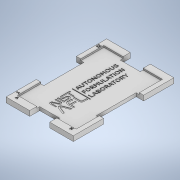
# Autodesk Inventor part: Thermal_underplate
Saved by Autodesk Inventor 2020 (Build 240168000, 168)
## iProperties
Created: 2021-08-09
Part Number: Thermal_underplate
Material: Generic
Document SubType Name: Modeling
Designer: pab2
Density: 1 g/cm^3
Appearance: Default
Author: pab2
Autodesk Inventor part; units mm, degrees
(part 1 of 3)
ref_plane "YZ Plane" through (0, 0, 0) normal (1, 0, 0) x (0, 1, 0)
ref_plane "XZ Plane" through (0, 0, 0) normal (0, 1, 0) x (-1, 0, 0)
ref_plane "XY Plane" through (0, 0, 0) normal (0, 0, 1) x (1, 0, 0)
sketch "Sketch1" plane through (0, 0, 0) normal (0, 1, 0) x (-1, 0, 0)
  line L0 (0, 0) -> (85.48, 0)
  line L1 (85.48, 0) -> (85.48, -127.76)
  line L2 (85.48, -127.76) -> (0, -127.76)
  line L3 (0, -127.76) -> (0, 0)
  line L4 (85.48, 0) -> (67.5195, -17.9605)
  line L5 (85.48, 0) -> (110.88, 0) construction
  line L6 (0, 0) -> (17.9605, -17.9605)
  line L7 (85.48, -127.76) -> (67.5195, -109.7995)
  line L8 (85.48, -127.76) -> (110.88, -127.76) construction
  line L9 (0, -127.76) -> (17.9605, -109.7995)
  line L10 (0, -127.76) -> (25.4, -127.76) construction
  dimension "d0" = 85.48
  dimension "d1" = 127.76
  dimension "d2" = 25.4
  dimension "d3" = 135
  dimension "d4" = 25.4
  dimension "d5" = 25.4
  dimension "d6" = 135
  dimension "d7" = 25.4
  dimension "d8" = 45
  constraints: 22 end point, 4 horizontal, 3 equal length, 2 parallel, 1 perpendicular
  measures "d0" distance of L1.end L2.end
  measures "d1" distance of L0.end L1.end
  measures "d2" distance of L0.end L4.end
  measures "d3" angle of L4 L5
  measures "d4" distance of L0.start L6.end
  measures "d5" distance of L1.end L7.end
  measures "d6" angle of L8 L7
  measures "d7" distance of L2.end L9.end
  measures "d8" angle of L10 L9
extrude "Extrusion1" add sketch "Sketch1" along normal blind 6.35
sketch "Sketch3" plane through (0, 6.35, 0) normal (0, 1, 0) x (1, 0, 0)
  line L0 (0, 127.76) -> (-85.48, 127.76) projected
  line L1 (-85.48, 127.76) -> (-85.48, 0) projected
  line L2 (-79.94, 9.08) -> (-5.54, 9.08)
  line L3 (-5.54, 9.08) -> (-5.54, 118.68)
  line L4 (-5.54, 118.68) -> (-79.94, 118.68)
  line L5 (-79.94, 118.68) -> (-79.94, 9.08)
  line L6 (-79.94, 9.08) -> (-5.54, 118.68) construction
  line L7 (-5.54, 9.08) -> (-79.94, 118.68) construction
  point P0 (0, 0)
  point P1 (-42.74, 127.76)
  point P2 (-85.48, 63.88)
  point P3 (-42.74, 63.88)
  dimension "d26" = 74.4
  dimension "d27" = 109.6
  constraints: 12 end point, 4 midpoint, 2 parallel, 1 horizontal, 1 perpendicular
  measures "d26" distance of L4.end L3.end
  measures "d27" distance of L3.end L2.end
extrude "Extrusion2" cut sketch "Sketch3" against normal blind 2
sketch "Sketch4" plane through (0, 0, 0) normal (0, -1, 0) x (1, 0, 0)
  line L0 (0, 0) -> (0, -127.76) projected
  line L1 (0, -127.76) -> (-85.48, -127.76) projected
  line L2 (-85.48, -127.76) -> (-85.48, 0) projected
  line L3 (-85.48, 0) -> (0, 0) projected
  line L4 (6.35, -38.48) -> (-6.35, -38.48)
  line L5 (-6.35, -38.48) -> (-6.35, -89.28)
  line L6 (-6.35, -89.28) -> (6.35, -89.28)
  line L7 (6.35, -89.28) -> (6.35, -38.48)
  line L8 (6.35, -38.48) -> (-6.35, -89.28) construction
  line L9 (-6.35, -38.48) -> (6.35, -89.28) construction
  line L10 (-55.44, -121.41) -> (-30.04, -121.41)
  line L11 (-30.04, -121.41) -> (-30.04, -134.11)
  line L12 (-30.04, -134.11) -> (-55.44, -134.11)
  line L13 (-55.44, -134.11) -> (-55.44, -121.41)
  line L14 (-55.44, -121.41) -> (-30.04, -134.11) construction
  line L15 (-30.04, -121.41) -> (-55.44, -134.11) construction
  line L16 (-79.13, -38.48) -> (-91.83, -38.48)
  line L17 (-91.83, -38.48) -> (-91.83, -89.28)
  line L18 (-91.83, -89.28) -> (-79.13, -89.28)
  line L19 (-79.13, -89.28) -> (-79.13, -38.48)
  line L20 (-79.13, -38.48) -> (-91.83, -89.28) construction
  line L21 (-91.83, -38.48) -> (-79.13, -89.28) construction
  line L22 (-55.44, 6.35) -> (-30.04, 6.35)
  line L23 (-30.04, 6.35) -> (-30.04, -6.35)
  line L24 (-30.04, -6.35) -> (-55.44, -6.35)
  line L25 (-55.44, -6.35) -> (-55.44, 6.35)
  line L26 (-55.44, 6.35) -> (-30.04, -6.35) construction
  line L27 (-30.04, 6.35) -> (-55.44, -6.35) construction
  line L28 (0, -38.48) -> (0, -89.28)
  line L29 (-30.04, -127.76) -> (-55.44, -127.76)
  line L30 (-85.48, -89.28) -> (-85.48, -38.48)
  line L31 (-55.44, 0) -> (-30.04, 0)
  line L32 (-6.35, -38.48) -> (0, -38.48)
  line L33 (0, -38.48) -> (0, -89.28)
  line L34 (0, -89.28) -> (-6.35, -89.28)
  line L35 (-6.35, -89.28) -> (-6.35, -38.48)
  line L36 (-30.04, -127.76) -> (-55.44, -127.76)
  line L37 (-55.44, -127.76) -> (-55.44, -121.41)
  line L38 (-55.44, -121.41) -> (-30.04, -121.41)
  line L39 (-30.04, -121.41) -> (-30.04, -127.76)
  line L40 (-85.48, -89.28) -> (-79.13, -89.28)
  line L41 (-79.13, -89.28) -> (-79.13, -38.48)
  line L42 (-79.13, -38.48) -> (-85.48, -38.48)
  line L43 (-85.48, -38.48) -> (-85.48, -89.28)
  line L44 (-55.44, -6.35) -> (-30.04, -6.35)
  line L45 (-30.04, -6.35) -> (-30.04, 0)
  line L46 (-30.04, 0) -> (-55.44, 0)
  line L47 (-55.44, 0) -> (-55.44, -6.35)
  line L48 (-30.04, -127.76) -> (-55.44, -127.76)
  line L49 (-55.44, -127.76) -> (-55.44, -115.0668)
  line L50 (-55.44, -115.0668) -> (-30.04, -115.0668)
  line L51 (-30.04, -115.0668) -> (-30.04, -127.76)
  line L52 (-55.44, 0) -> (-30.04, 0)
  line L53 (-30.04, 0) -> (-30.04, -12.7)
  line L54 (-30.04, -12.7) -> (-55.44, -12.7)
  line L55 (-55.44, -12.7) -> (-55.44, 0)
  line L56 (-85.48, -38.48) -> (-75.955, -38.48)
  line L57 (-75.955, -38.48) -> (-75.955, -89.28)
  line L58 (-75.955, -89.28) -> (-85.48, -89.28)
  line L59 (-85.48, -89.28) -> (-85.48, -38.48)
  line L60 (0, -89.28) -> (-9.525, -89.28)
  line L61 (-9.525, -89.28) -> (-9.525, -38.48)
  line L62 (-9.525, -38.48) -> (0, -38.48)
  line L63 (0, -38.48) -> (0, -89.28)
  point P0 (0, -63.88)
  point P1 (-42.74, -127.76)
  point P2 (-85.48, -63.88)
  point P3 (-42.74, 0)
  dimension "d30" = 12.7
  dimension "d31" = 50.8
  dimension "d32" = 25.4
  dimension "d33" = 12.7
  dimension "d34" = 12.7
  dimension "d35" = 50.8
  dimension "d36" = 25.4
  dimension "d37" = 12.7
  dimension "d40" = 12.7
  dimension "d41" = 9.525
  dimension "d42" = 50.8
  dimension "d43" = 9.525
  constraints: 120 end point, 24 parallel, 20 midpoint, 12 horizontal, 12 perpendicular, 2 point on line
  measures "d30" distance of L6.end L5.end
  measures "d31" distance of L5.end L4.end
  measures "d32" distance of L11.end L12.end
  measures "d33" distance of L10.end L11.end
  measures "d34" distance of L18.end L17.end
  measures "d35" distance of L17.end L16.end
  measures "d36" distance of L23.end L24.end
  measures "d37" distance of L22.end L23.end
  measures "d40" distance of L52.end L53.end
  measures "d41" distance of L57.end L58.end
  measures "d42" distance of L56.end L57.end
  measures "d43" distance of L61.end L62.end
extrude "Extrusion3" cut sketch "Sketch4" against normal blind 12.7 contours L0 L6 L5 L4 | L23 L24 L25 L3 | L5 L60 L61 L62 | L53 L54 L55 L24 | L1 L13 L10 L11 | L16 L19 L18 L2 | L10 L49 L50 L51 | L56 L57 L58 L19
sketch "Sketch5" plane through (0, 6.35, 0) normal (0, 1, 0) x (1, 0, 0)
  line L0 (-84.169, 11.0386) -> (-84.169, 16.2129) construction
  line L1 (-84.169, 16.2129) -> (-77.0974, 16.2129) construction
  line L2 (-77.0974, 16.2129) -> (-77.0974, 11.0386) construction
  line L3 (-77.0974, 11.0386) -> (-84.169, 11.0386) construction
  line L4 (-78.4772, 7.4165) -> (-71.4056, 7.4165) construction
  line L5 (-71.4056, 7.4165) -> (-71.4056, 2.9321) construction
  line L6 (-71.4056, 2.9321) -> (-78.4772, 2.9321) construction
  line L7 (-78.4772, 2.9321) -> (-78.4772, 7.4165) construction
  line L8 (-84.1338, 112.1455) -> (-84.1338, 117.3198) construction
  line L9 (-84.1338, 117.3198) -> (-77.0622, 117.3198) construction
  line L10 (-77.0622, 117.3198) -> (-77.0622, 112.1455) construction
  line L11 (-77.0622, 112.1455) -> (-84.1338, 112.1455) construction
  line L12 (-10.3281, 7.9734) -> (-3.2565, 7.9734) construction
  line L13 (-3.2565, 7.9734) -> (-3.2565, 3.489) construction
  line L14 (-3.2565, 3.489) -> (-10.3281, 3.489) construction
  line L15 (-10.3281, 3.489) -> (-10.3281, 7.9734) construction
  line L16 (-81.1111, 12.9874) -> (-81.1111, 11.5004)
  line L17 (-81.1111, 11.5004) -> (-81.4223, 11.5004)
  line L18 (-81.4223, 11.5004) -> (-81.4223, 12.0537)
  line L19 (-81.4223, 12.0537) -> (-83.465, 12.0537)
  line L20 (-83.465, 12.0537) -> (-83.465, 11.5004)
  line L21 (-83.465, 11.5004) -> (-83.7441, 11.5004)
  spline S0 degree 2 poles (-83.7441, 11.5004) (-83.7441, 11.8141) (-83.922, 12.1105) (-84.169, 12.1303) knots 0 0 0 1 2 2 2
  line L22 (-84.169, 12.1303) -> (-84.169, 12.4465)
  line L23 (-84.169, 12.4465) -> (-81.4223, 12.4465)
  line L24 (-81.4223, 12.4465) -> (-81.4223, 12.9874)
  line L25 (-81.4223, 12.9874) -> (-81.1111, 12.9874)
  line L26 (-81.0215, 114.0943) -> (-81.0215, 112.6074)
  line L27 (-81.0215, 112.6074) -> (-81.3328, 112.6074)
  line L28 (-81.3328, 112.6074) -> (-81.3328, 113.1607)
  line L29 (-81.3328, 113.1607) -> (-83.3755, 113.1607)
  line L30 (-83.3755, 113.1607) -> (-83.3755, 112.6074)
  line L31 (-83.3755, 112.6074) -> (-83.6546, 112.6074)
  spline S1 degree 2 poles (-83.6546, 112.6074) (-83.6546, 112.9211) (-83.8324, 113.2175) (-84.0794, 113.2372) knots 0 0 0 1 2 2 2
  line L32 (-84.0794, 113.2372) -> (-84.0794, 113.5534)
  line L33 (-84.0794, 113.5534) -> (-81.3328, 113.5534)
  line L34 (-81.3328, 113.5534) -> (-81.3328, 114.0943)
  line L35 (-81.3328, 114.0943) -> (-81.0215, 114.0943)
  line L36 (-81.0215, 116.5347) -> (-81.0215, 114.655)
  line L37 (-81.0215, 114.655) -> (-81.4538, 114.655)
  spline S2 degree 2 poles (-81.4538, 114.655) (-81.644, 114.8576) (-81.9972, 115.2182) (-82.1874, 115.3911) knots 0 0 0 1 2 2 2
  spline S3 degree 2 poles (-82.1874, 115.3911) (-82.5702, 115.7394) (-83.0297, 115.9938) (-83.2742, 115.9938) knots 0 0 0 1 2 2 2
  spline S4 degree 2 poles (-83.2742, 115.9938) (-83.4026, 115.9938) (-83.5953, 115.9147) (-83.657, 115.8431) knots 0 0 0 1 2 2 2
  spline S5 degree 2 poles (-83.657, 115.8431) (-83.7188, 115.7715) (-83.7805, 115.5838) (-83.7805, 115.4701) knots 0 0 0 1 2 2 2
  spline S6 degree 2 poles (-83.7805, 115.4701) (-83.7805, 115.3615) (-83.7262, 115.1392) (-83.6842, 115.0379) knots 0 0 0 1 2 2 2
  spline S7 degree 2 poles (-83.6842, 115.0379) (-83.6496, 114.9514) (-83.5508, 114.7909) (-83.5163, 114.7415) knots 0 0 0 1 2 2 2
  line L38 (-83.5163, 114.7415) -> (-83.5163, 114.7193)
  line L39 (-83.5163, 114.7193) -> (-83.951, 114.7193)
  spline S8 degree 2 poles (-83.951, 114.7193) (-84.0127, 114.8452) (-84.1338, 115.2972) (-84.1338, 115.4998) knots 0 0 0 1 2 2 2
  spline S9 degree 2 poles (-84.1338, 115.4998) (-84.1338, 115.9271) (-83.6817, 116.4087) (-83.2964, 116.4087) knots 0 0 0 1 2 2 2
  spline S10 degree 2 poles (-83.2964, 116.4087) (-83.1161, 116.4087) (-82.8148, 116.3248) (-82.6863, 116.2507) knots 0 0 0 1 2 2 2
  spline S11 degree 2 poles (-82.6863, 116.2507) (-82.553, 116.1766) (-82.2911, 115.9617) (-82.1652, 115.8431) knots 0 0 0 1 2 2 2
  spline S12 degree 2 poles (-82.1652, 115.8431) (-81.9552, 115.6505) (-81.5057, 115.1787) (-81.3748, 115.0379) knots 0 0 0 1 2 2 2
  line L40 (-81.3748, 115.0379) -> (-81.3748, 116.5347)
  line L41 (-81.3748, 116.5347) -> (-81.0215, 116.5347)
  line L42 (-7.8062, 4.9254) -> (-8.2113, 4.9254)
  line L43 (-8.2113, 4.9254) -> (-8.2113, 6.4173)
  line L44 (-8.2113, 6.4173) -> (-9.6143, 6.4173)
  line L45 (-9.6143, 6.4173) -> (-9.6143, 4.9254)
  line L46 (-9.6143, 4.9254) -> (-10.0194, 4.9254)
  line L47 (-10.0194, 4.9254) -> (-10.0194, 7.9734)
  line L48 (-10.0194, 7.9734) -> (-9.6143, 7.9734)
  line L49 (-9.6143, 7.9734) -> (-9.6143, 6.7779)
  line L50 (-9.6143, 6.7779) -> (-8.2113, 6.7779)
  line L51 (-8.2113, 6.7779) -> (-8.2113, 7.9734)
  line L52 (-8.2113, 7.9734) -> (-7.8062, 7.9734)
  line L53 (-7.8062, 7.9734) -> (-7.8062, 4.9254)
  line L54 (-78.497, 4.3685) -> (-77.4694, 7.4165)
  line L55 (-77.4694, 7.4165) -> (-76.9705, 7.4165)
  line L56 (-76.9705, 7.4165) -> (-75.943, 4.3685)
  line L57 (-75.943, 4.3685) -> (-76.3703, 4.3685)
  line L58 (-76.3703, 4.3685) -> (-76.6469, 5.2207)
  line L59 (-76.6469, 5.2207) -> (-77.8103, 5.2207)
  line L60 (-77.8103, 5.2207) -> (-78.0869, 4.3685)
  line L61 (-78.0869, 4.3685) -> (-78.497, 4.3685)
  line L62 (-76.7581, 5.5665) -> (-77.2299, 7.0016)
  line L63 (-77.2299, 7.0016) -> (-77.6992, 5.5665)
  line L64 (-77.6992, 5.5665) -> (-76.7581, 5.5665)
  point P0 (0, 0)
  constraints: 8 other
extrude "Extrusion4" add sketch "Sketch5" along normal blind 0.5
sketch "Sketch6" plane through (0, 4.35, 0) normal (0, 1, 0) x (1, 0, 0)
  line L0 (-31.536, 53.5393) -> (-31.536, 52.6573)
  line L1 (-31.536, 52.6573) -> (-54.4666, 52.6573)
  line L2 (-54.4666, 52.6573) -> (-54.4666, 53.5393)
  line L3 (-54.4666, 53.5393) -> (-31.536, 53.5393)
  line L4 (-32.8598, 21.4412) -> (-32.8598, 19.3775)
  line L5 (-32.8598, 19.3775) -> (-42.3845, 23.1397)
  spline S0 degree 3 poles (-42.3845, 23.1397) (-43.3845, 23.5366) (-43.7655, 24.2668) (-43.7655, 25.3938) (-43.7655, 26.505) (-43.3845, 27.2353) (-42.3845, 27.6163) knots 2 2 2 2 3 3 3 4 4 4 4
  line L6 (-42.3845, 23.1397) -> (-43.3845, 23.5366) construction
  line L7 (-43.3845, 23.5366) -> (-43.7655, 24.2668) construction
  line L8 (-43.7655, 24.2668) -> (-43.7655, 25.3938) construction
  line L9 (-43.7655, 25.3938) -> (-43.7655, 26.505) construction
  line L10 (-43.7655, 26.505) -> (-43.3845, 27.2353) construction
  line L11 (-43.3845, 27.2353) -> (-42.3845, 27.6163) construction
  line L12 (-42.3845, 27.6163) -> (-32.8598, 31.2356)
  line L13 (-32.8598, 31.2356) -> (-32.8598, 29.156)
  line L14 (-32.8598, 29.156) -> (-41.4796, 25.9018)
  spline S1 degree 3 poles (-41.4796, 25.9018) (-41.7337, 25.8065) (-41.8448, 25.632) (-41.8448, 25.378) (-41.8448, 25.124) (-41.7337, 24.9494) (-41.4796, 24.8382) knots 7 7 7 7 8 8 8 9 9 9 9
  line L15 (-41.4796, 25.9018) -> (-41.7337, 25.8065) construction
  line L16 (-41.7337, 25.8065) -> (-41.8448, 25.632) construction
  line L17 (-41.8448, 25.632) -> (-41.8448, 25.378) construction
  line L18 (-41.8448, 25.378) -> (-41.8448, 25.124) construction
  line L19 (-41.8448, 25.124) -> (-41.7337, 24.9494) construction
  line L20 (-41.7337, 24.9494) -> (-41.4796, 24.8382) construction
  line L21 (-41.4796, 24.8382) -> (-32.8598, 21.4412)
  line L22 (-43.575, 41.1258) -> (-41.7018, 41.1258)
  line L23 (-41.7018, 41.1258) -> (-41.7018, 36.8079)
  spline S2 degree 3 poles (-41.7018, 36.8079) (-41.7018, 35.1094) (-40.8922, 34.6014) (-39.8921, 34.6014) knots 2 2 2 2 3 3 3 3
  line L24 (-41.7018, 36.8079) -> (-41.7018, 35.1094) construction
  line L25 (-41.7018, 35.1094) -> (-40.8922, 34.6014) construction
  line L26 (-40.8922, 34.6014) -> (-39.8921, 34.6014) construction
  line L27 (-39.8921, 34.6014) -> (-38.8761, 34.6014)
  line L28 (-38.8761, 34.6014) -> (-38.8761, 41.0623)
  line L29 (-38.8761, 41.0623) -> (-37.0983, 41.0623)
  line L30 (-37.0983, 41.0623) -> (-37.0983, 34.6014)
  line L31 (-37.0983, 34.6014) -> (-32.8598, 34.6014)
  line L32 (-32.8598, 34.6014) -> (-32.8598, 32.7283)
  line L33 (-32.8598, 32.7283) -> (-39.8763, 32.7283)
  spline S3 degree 3 poles (-39.8763, 32.7283) (-42.0193, 32.7283) (-43.575, 33.8395) (-43.575, 36.681) knots 10 10 10 10 11 11 11 11
  line L34 (-39.8763, 32.7283) -> (-42.0193, 32.7283) construction
  line L35 (-42.0193, 32.7283) -> (-43.575, 33.8395) construction
  line L36 (-43.575, 33.8395) -> (-43.575, 36.681) construction
  line L37 (-43.575, 36.681) -> (-43.575, 41.1258)
  line L38 (-43.575, 45.1105) -> (-36.5745, 45.1105)
  spline S4 degree 3 poles (-36.5745, 45.1105) (-35.5427, 45.1105) (-34.7331, 45.6185) (-34.7331, 47.3012) knots 1 1 1 1 2 2 2 2
  line L39 (-36.5745, 45.1105) -> (-35.5427, 45.1105) construction
  line L40 (-35.5427, 45.1105) -> (-34.7331, 45.6185) construction
  line L41 (-34.7331, 45.6185) -> (-34.7331, 47.3012) construction
  line L42 (-34.7331, 47.3012) -> (-34.7331, 51.4603)
  line L43 (-34.7331, 51.4603) -> (-32.8598, 51.4603)
  line L44 (-32.8598, 51.4603) -> (-32.8598, 47.1901)
  spline S5 degree 3 poles (-32.8598, 47.1901) (-32.8598, 44.3486) (-34.4156, 43.2373) (-36.5586, 43.2373) knots 5 5 5 5 6 6 6 6
  line L45 (-32.8598, 47.1901) -> (-32.8598, 44.3486) construction
  line L46 (-32.8598, 44.3486) -> (-34.4156, 43.2373) construction
  line L47 (-34.4156, 43.2373) -> (-36.5586, 43.2373) construction
  line L48 (-36.5586, 43.2373) -> (-43.575, 43.2373)
  line L49 (-43.575, 43.2373) -> (-43.575, 45.1105)
  line L50 (-44.8529, 23.7071) -> (-44.8529, 22.2084)
  line L51 (-44.8529, 22.2084) -> (-51.7114, 22.2084)
  spline S6 degree 3 poles (-51.7114, 22.2084) (-52.8291, 22.2084) (-53.5785, 22.8434) (-53.5785, 24.1771) (-53.5785, 25.371) (-52.9689, 25.9044) (-51.9908, 26.2601) knots 2 2 2 2 3 3 3 4 4 4 4
  line L52 (-51.7114, 22.2084) -> (-52.8291, 22.2084) construction
  line L53 (-52.8291, 22.2084) -> (-53.5785, 22.8434) construction
  line L54 (-53.5785, 22.8434) -> (-53.5785, 24.1771) construction
  line L55 (-53.5785, 24.1771) -> (-53.5785, 25.371) construction
  line L56 (-53.5785, 25.371) -> (-52.9689, 25.9044) construction
  line L57 (-52.9689, 25.9044) -> (-51.9908, 26.2601) construction
  line L58 (-51.9908, 26.2601) -> (-46.5167, 28.7622)
  spline S7 degree 3 poles (-46.5167, 28.7622) (-46.3135, 28.8638) (-46.1611, 29.0289) (-46.1611, 29.3083) (-46.1611, 29.6259) (-46.3516, 29.8164) (-46.6437, 29.8164) knots 5 5 5 5 6 6 6 7 7 7 7
  line L59 (-46.5167, 28.7622) -> (-46.3135, 28.8638) construction
  line L60 (-46.3135, 28.8638) -> (-46.1611, 29.0289) construction
  line L61 (-46.1611, 29.0289) -> (-46.1611, 29.3083) construction
  line L62 (-46.1611, 29.3083) -> (-46.1611, 29.6259) construction
  line L63 (-46.1611, 29.6259) -> (-46.3516, 29.8164) construction
  line L64 (-46.3516, 29.8164) -> (-46.6437, 29.8164) construction
  line L65 (-46.6437, 29.8164) -> (-53.4261, 29.8164)
  line L66 (-53.4261, 29.8164) -> (-53.4261, 31.3278)
  line L67 (-53.4261, 31.3278) -> (-46.5802, 31.3278)
  spline S8 degree 3 poles (-46.5802, 31.3278) (-45.4498, 31.3278) (-44.7004, 30.6801) (-44.7004, 29.3591) (-44.7004, 28.1652) (-45.3101, 27.6191) (-46.2881, 27.2635) knots 10 10 10 10 11 11 11 12 12 12 12
  line L68 (-46.5802, 31.3278) -> (-45.4498, 31.3278) construction
  line L69 (-45.4498, 31.3278) -> (-44.7004, 30.6801) construction
  line L70 (-44.7004, 30.6801) -> (-44.7004, 29.3591) construction
  line L71 (-44.7004, 29.3591) -> (-44.7004, 28.1652) construction
  line L72 (-44.7004, 28.1652) -> (-45.3101, 27.6191) construction
  line L73 (-45.3101, 27.6191) -> (-46.2881, 27.2635) construction
  line L74 (-46.2881, 27.2635) -> (-51.7623, 24.7613)
  spline S9 degree 3 poles (-51.7623, 24.7613) (-52.0163, 24.647) (-52.1306, 24.4946) (-52.1306, 24.2278) (-52.1306, 23.885) (-51.9401, 23.7071) (-51.6352, 23.7071) knots 13 13 13 13 14 14 14 15 15 15 15
  line L75 (-51.7623, 24.7613) -> (-52.0163, 24.647) construction
  line L76 (-52.0163, 24.647) -> (-52.1306, 24.4946) construction
  line L77 (-52.1306, 24.4946) -> (-52.1306, 24.2278) construction
  line L78 (-52.1306, 24.2278) -> (-52.1306, 23.885) construction
  line L79 (-52.1306, 23.885) -> (-51.9401, 23.7071) construction
  line L80 (-51.9401, 23.7071) -> (-51.6352, 23.7071) construction
  line L81 (-51.6352, 23.7071) -> (-44.8529, 23.7071)
  line L82 (-53.5384, 34.4015) -> (-44.9652, 34.4015)
  line L83 (-44.9652, 34.4015) -> (-44.9652, 32.9027)
  line L84 (-44.9652, 32.9027) -> (-53.5384, 32.9027)
  line L85 (-53.5384, 32.9027) -> (-53.5384, 34.4015)
  line L86 (-53.5384, 42.2674) -> (-52.0397, 42.2674)
  line L87 (-52.0397, 42.2674) -> (-52.0397, 37.8727)
  spline S10 degree 3 poles (-52.0397, 37.8727) (-52.0397, 37.098) (-51.6206, 36.7551) (-51.0236, 36.7551) (-50.5028, 36.7551) (-50.0075, 37.0218) (-50.0075, 38.0252) knots 2 2 2 2 3 3 3 4 4 4 4
  line L88 (-52.0397, 37.8727) -> (-52.0397, 37.098) construction
  line L89 (-52.0397, 37.098) -> (-51.6206, 36.7551) construction
  line L90 (-51.6206, 36.7551) -> (-51.0236, 36.7551) construction
  line L91 (-51.0236, 36.7551) -> (-50.5028, 36.7551) construction
  line L92 (-50.5028, 36.7551) -> (-50.0075, 37.0218) construction
  line L93 (-50.0075, 37.0218) -> (-50.0075, 38.0252) construction
  line L94 (-50.0075, 38.0252) -> (-50.0075, 40.0319)
  spline S11 degree 3 poles (-50.0075, 40.0319) (-50.0075, 42.3689) (-48.712, 42.9151) (-47.48, 42.9151) (-46.032, 42.9151) (-44.9652, 42.1403) (-44.9652, 40.1844) knots 5 5 5 5 6 6 6 7 7 7 7
  line L95 (-50.0075, 40.0319) -> (-50.0075, 42.3689) construction
  line L96 (-50.0075, 42.3689) -> (-48.712, 42.9151) construction
  line L97 (-48.712, 42.9151) -> (-47.48, 42.9151) construction
  line L98 (-47.48, 42.9151) -> (-46.032, 42.9151) construction
  line L99 (-46.032, 42.9151) -> (-44.9652, 42.1403) construction
  line L100 (-44.9652, 42.1403) -> (-44.9652, 40.1844) construction
  line L101 (-44.9652, 40.1844) -> (-44.9652, 35.4088)
  line L102 (-44.9652, 35.4088) -> (-46.4639, 35.4088)
  line L103 (-46.4639, 35.4088) -> (-46.4639, 40.2352)
  spline S12 degree 3 poles (-46.4639, 40.2352) (-46.4639, 41.0481) (-46.9085, 41.4164) (-47.5308, 41.4164) (-48.0896, 41.4164) (-48.5977, 41.1242) (-48.5977, 40.0701) knots 10 10 10 10 11 11 11 12 12 12 12
  line L104 (-46.4639, 40.2352) -> (-46.4639, 41.0481) construction
  line L105 (-46.4639, 41.0481) -> (-46.9085, 41.4164) construction
  line L106 (-46.9085, 41.4164) -> (-47.5308, 41.4164) construction
  line L107 (-47.5308, 41.4164) -> (-48.0896, 41.4164) construction
  line L108 (-48.0896, 41.4164) -> (-48.5977, 41.1242) construction
  line L109 (-48.5977, 41.1242) -> (-48.5977, 40.0701) construction
  line L110 (-48.5977, 40.0701) -> (-48.5977, 38.076)
  spline S13 degree 3 poles (-48.5977, 38.076) (-48.5977, 35.7898) (-49.8805, 35.2564) (-51.0744, 35.2564) (-52.4969, 35.2564) (-53.5384, 36.0184) (-53.5384, 37.9235) knots 13 13 13 13 14 14 14 15 15 15 15
  line L111 (-48.5977, 38.076) -> (-48.5977, 35.7898) construction
  line L112 (-48.5977, 35.7898) -> (-49.8805, 35.2564) construction
  line L113 (-49.8805, 35.2564) -> (-51.0744, 35.2564) construction
  line L114 (-51.0744, 35.2564) -> (-52.4969, 35.2564) construction
  line L115 (-52.4969, 35.2564) -> (-53.5384, 36.0184) construction
  line L116 (-53.5384, 36.0184) -> (-53.5384, 37.9235) construction
  line L117 (-53.5384, 37.9235) -> (-53.5384, 42.2674)
  line L118 (-53.5384, 48.7753) -> (-52.0397, 48.7753)
  line L119 (-52.0397, 48.7753) -> (-52.0397, 46.2733)
  line L120 (-52.0397, 46.2733) -> (-44.9652, 46.2733)
  line L121 (-44.9652, 46.2733) -> (-44.9652, 44.7618)
  line L122 (-44.9652, 44.7618) -> (-52.0397, 44.7618)
  line L123 (-52.0397, 44.7618) -> (-52.0397, 42.2597)
  line L124 (-52.0397, 42.2597) -> (-53.5384, 42.2597)
  line L125 (-53.5384, 42.2597) -> (-53.5384, 48.7753)
  line L126 (-50.7059, 56.687) -> (-49.81, 56.3202)
  spline S14 degree 3 poles (-49.81, 56.3202) (-49.6195, 56.2426) (-49.5208, 56.1227) (-49.5208, 55.9392) (-49.5208, 55.7135) (-49.6689, 55.5583) (-49.8735, 55.5442) knots 1 1 1 1 2 2 2 3 3 3 3
  line L127 (-49.81, 56.3202) -> (-49.6195, 56.2426) construction
  line L128 (-49.6195, 56.2426) -> (-49.5208, 56.1227) construction
  line L129 (-49.5208, 56.1227) -> (-49.5208, 55.9392) construction
  line L130 (-49.5208, 55.9392) -> (-49.5208, 55.7135) construction
  line L131 (-49.5208, 55.7135) -> (-49.6689, 55.5583) construction
  line L132 (-49.6689, 55.5583) -> (-49.8735, 55.5442) construction
  spline S15 degree 3 poles (-49.8735, 55.5442) (-49.9652, 55.5372) (-50.0499, 55.5654) (-50.1486, 55.6077) knots 3 3 3 3 4 4 4 4
  line L133 (-49.8735, 55.5442) -> (-49.9652, 55.5372) construction
  line L134 (-49.9652, 55.5372) -> (-50.0499, 55.5654) construction
  line L135 (-50.0499, 55.5654) -> (-50.1486, 55.6077) construction
  line L136 (-50.1486, 55.6077) -> (-53.7111, 57.0891)
  spline S16 degree 3 poles (-53.7111, 57.0891) (-54.1061, 57.2443) (-54.2543, 57.4559) (-54.2543, 57.7734) knots 5 5 5 5 6 6 6 6
  line L137 (-53.7111, 57.0891) -> (-54.1061, 57.2443) construction
  line L138 (-54.1061, 57.2443) -> (-54.2543, 57.4559) construction
  line L139 (-54.2543, 57.4559) -> (-54.2543, 57.7734) construction
  line L140 (-54.2543, 57.7734) -> (-54.2543, 57.8228)
  spline S17 degree 3 poles (-54.2543, 57.8228) (-54.2543, 58.1473) (-54.1061, 58.3518) (-53.7111, 58.5141) knots 7 7 7 7 8 8 8 8
  line L141 (-54.2543, 57.8228) -> (-54.2543, 58.1473) construction
  line L142 (-54.2543, 58.1473) -> (-54.1061, 58.3518) construction
  line L143 (-54.1061, 58.3518) -> (-53.7111, 58.5141) construction
  line L144 (-53.7111, 58.5141) -> (-50.1204, 59.9955)
  spline S18 degree 3 poles (-50.1204, 59.9955) (-50.0287, 60.0308) (-49.9511, 60.052) (-49.8947, 60.052) (-49.676, 60.052) (-49.5208, 59.8756) (-49.5208, 59.6428) (-49.5208, 59.4735) (-49.6266, 59.3324) (-49.8171, 59.2548) knots 9 9 9 9 10 10 10 11 11 11 12 12 12 12
  line L145 (-50.1204, 59.9955) -> (-50.0287, 60.0308) construction
  line L146 (-50.0287, 60.0308) -> (-49.9511, 60.052) construction
  line L147 (-49.9511, 60.052) -> (-49.8947, 60.052) construction
  line L148 (-49.8947, 60.052) -> (-49.676, 60.052) construction
  line L149 (-49.676, 60.052) -> (-49.5208, 59.8756) construction
  line L150 (-49.5208, 59.8756) -> (-49.5208, 59.6428) construction
  line L151 (-49.5208, 59.6428) -> (-49.5208, 59.4735) construction
  line L152 (-49.5208, 59.4735) -> (-49.6266, 59.3324) construction
  line L153 (-49.6266, 59.3324) -> (-49.8171, 59.2548) construction
  line L154 (-49.8171, 59.2548) -> (-50.7059, 58.8951)
  line L155 (-50.7059, 58.8951) -> (-50.7059, 56.687)
  line L156 (-51.4114, 58.62) -> (-53.4783, 57.8086)
  line L157 (-53.4783, 57.8086) -> (-53.4783, 57.7875)
  line L158 (-53.4783, 57.7875) -> (-51.4114, 56.9551)
  line L159 (-51.4114, 56.9551) -> (-51.4114, 58.62)
  spline S19 degree 3 poles (-50.2332, 62.8958) (-50.2332, 63.6506) (-50.7482, 64.1232) (-51.5525, 64.1232) knots 0 0 0 0 1 1 1 1
  line L160 (-50.2332, 62.8958) -> (-50.2332, 63.6506) construction
  line L161 (-50.2332, 63.6506) -> (-50.7482, 64.1232) construction
  line L162 (-50.7482, 64.1232) -> (-51.5525, 64.1232) construction
  line L163 (-51.5525, 64.1232) -> (-53.9156, 64.1232)
  spline S20 degree 3 poles (-53.9156, 64.1232) (-54.1203, 64.1232) (-54.2613, 64.2854) (-54.2613, 64.5112) (-54.2613, 64.7369) (-54.1203, 64.8992) (-53.9156, 64.8992) knots 2 2 2 2 3 3 3 4 4 4 4
  line L164 (-53.9156, 64.1232) -> (-54.1203, 64.1232) construction
  line L165 (-54.1203, 64.1232) -> (-54.2613, 64.2854) construction
  line L166 (-54.2613, 64.2854) -> (-54.2613, 64.5112) construction
  line L167 (-54.2613, 64.5112) -> (-54.2613, 64.7369) construction
  line L168 (-54.2613, 64.7369) -> (-54.1203, 64.8992) construction
  line L169 (-54.1203, 64.8992) -> (-53.9156, 64.8992) construction
  line L170 (-53.9156, 64.8992) -> (-51.5101, 64.8992)
  spline S21 degree 3 poles (-51.5101, 64.8992) (-50.3391, 64.8992) (-49.4784, 64.1514) (-49.4784, 62.8958) (-49.4784, 61.633) (-50.3391, 60.8923) (-51.5101, 60.8923) knots 5 5 5 5 6 6 6 7 7 7 7
  line L171 (-51.5101, 64.8992) -> (-50.3391, 64.8992) construction
  line L172 (-50.3391, 64.8992) -> (-49.4784, 64.1514) construction
  line L173 (-49.4784, 64.1514) -> (-49.4784, 62.8958) construction
  line L174 (-49.4784, 62.8958) -> (-49.4784, 61.633) construction
  line L175 (-49.4784, 61.633) -> (-50.3391, 60.8923) construction
  line L176 (-50.3391, 60.8923) -> (-51.5101, 60.8923) construction
  line L177 (-51.5101, 60.8923) -> (-53.9156, 60.8923)
  spline S22 degree 3 poles (-53.9156, 60.8923) (-54.1203, 60.8923) (-54.2613, 61.0545) (-54.2613, 61.2803) (-54.2613, 61.506) (-54.1203, 61.6683) (-53.9156, 61.6683) knots 8 8 8 8 9 9 9 10 10 10 10
  line L178 (-53.9156, 60.8923) -> (-54.1203, 60.8923) construction
  line L179 (-54.1203, 60.8923) -> (-54.2613, 61.0545) construction
  line L180 (-54.2613, 61.0545) -> (-54.2613, 61.2803) construction
  line L181 (-54.2613, 61.2803) -> (-54.2613, 61.506) construction
  line L182 (-54.2613, 61.506) -> (-54.1203, 61.6683) construction
  line L183 (-54.1203, 61.6683) -> (-53.9156, 61.6683) construction
  line L184 (-53.9156, 61.6683) -> (-51.5525, 61.6683)
  spline S23 degree 3 poles (-51.5525, 61.6683) (-50.7553, 61.6683) (-50.2332, 62.1339) (-50.2332, 62.8958) knots 11 11 11 11 12 12 12 12
  line L185 (-51.5525, 61.6683) -> (-50.7553, 61.6683) construction
  line L186 (-50.7553, 61.6683) -> (-50.2332, 62.1339) construction
  line L187 (-50.2332, 62.1339) -> (-50.2332, 62.8958) construction
  spline S24 degree 3 poles (-53.8521, 65.6479) (-54.0779, 65.6479) (-54.2119, 65.796) (-54.2119, 66.0288) knots 0 0 0 0 1 1 1 1
  line L188 (-53.8521, 65.6479) -> (-54.0779, 65.6479) construction
  line L189 (-54.0779, 65.6479) -> (-54.2119, 65.796) construction
  line L190 (-54.2119, 65.796) -> (-54.2119, 66.0288) construction
  line L191 (-54.2119, 66.0288) -> (-54.2119, 69.6336)
  spline S25 degree 3 poles (-54.2119, 69.6336) (-54.2119, 69.8663) (-54.0779, 70.0074) (-53.8521, 70.0074) (-53.6335, 70.0074) (-53.4995, 69.8663) (-53.4995, 69.6336) knots 2 2 2 2 3 3 3 4 4 4 4
  line L192 (-54.2119, 69.6336) -> (-54.2119, 69.8663) construction
  line L193 (-54.2119, 69.8663) -> (-54.0779, 70.0074) construction
  line L194 (-54.0779, 70.0074) -> (-53.8521, 70.0074) construction
  line L195 (-53.8521, 70.0074) -> (-53.6335, 70.0074) construction
  line L196 (-53.6335, 70.0074) -> (-53.4995, 69.8663) construction
  line L197 (-53.4995, 69.8663) -> (-53.4995, 69.6336) construction
  line L198 (-53.4995, 69.6336) -> (-53.4995, 68.2226)
  line L199 (-53.4995, 68.2226) -> (-49.8664, 68.2226)
  spline S26 degree 3 poles (-49.8664, 68.2226) (-49.6619, 68.2226) (-49.5208, 68.0604) (-49.5208, 67.8347) (-49.5208, 67.6089) (-49.6619, 67.4466) (-49.8664, 67.4466) knots 6 6 6 6 7 7 7 8 8 8 8
  line L200 (-49.8664, 68.2226) -> (-49.6619, 68.2226) construction
  line L201 (-49.6619, 68.2226) -> (-49.5208, 68.0604) construction
  line L202 (-49.5208, 68.0604) -> (-49.5208, 67.8347) construction
  line L203 (-49.5208, 67.8347) -> (-49.5208, 67.6089) construction
  line L204 (-49.5208, 67.6089) -> (-49.6619, 67.4466) construction
  line L205 (-49.6619, 67.4466) -> (-49.8664, 67.4466) construction
  line L206 (-49.8664, 67.4466) -> (-53.4995, 67.4466)
  line L207 (-53.4995, 67.4466) -> (-53.4995, 66.0217)
  spline S27 degree 3 poles (-53.4995, 66.0217) (-53.4995, 65.796) (-53.6335, 65.6479) (-53.8521, 65.6479) knots 10 10 10 10 11 11 11 11
  line L208 (-53.4995, 66.0217) -> (-53.4995, 65.796) construction
  line L209 (-53.4995, 65.796) -> (-53.6335, 65.6479) construction
  line L210 (-53.6335, 65.6479) -> (-53.8521, 65.6479) construction
  spline S28 degree 3 poles (-51.8981, 70.2339) (-53.2878, 70.2339) (-54.2895, 71.3062) (-54.2895, 72.7028) (-54.2895, 74.0996) (-53.2878, 75.179) (-51.8981, 75.179) (-50.5014, 75.179) (-49.4925, 74.0996) (-49.4925, 72.7028) (-49.4925, 71.3062) (-50.5014, 70.2339) (-51.8981, 70.2339) knots 0 0 0 0 1 1 1 2 2 2 3 3 3 4 4 4 4
  line L211 (-51.8981, 70.2339) -> (-53.2878, 70.2339) construction
  line L212 (-53.2878, 70.2339) -> (-54.2895, 71.3062) construction
  line L213 (-54.2895, 71.3062) -> (-54.2895, 72.7028) construction
  line L214 (-54.2895, 72.7028) -> (-54.2895, 74.0996) construction
  line L215 (-54.2895, 74.0996) -> (-53.2878, 75.179) construction
  line L216 (-53.2878, 75.179) -> (-51.8981, 75.179) construction
  line L217 (-51.8981, 75.179) -> (-50.5014, 75.179) construction
  line L218 (-50.5014, 75.179) -> (-49.4925, 74.0996) construction
  line L219 (-49.4925, 74.0996) -> (-49.4925, 72.7028) construction
  line L220 (-49.4925, 72.7028) -> (-49.4925, 71.3062) construction
  line L221 (-49.4925, 71.3062) -> (-50.5014, 70.2339) construction
  line L222 (-50.5014, 70.2339) -> (-51.8981, 70.2339) construction
  spline S29 degree 3 poles (-50.2544, 72.7028) (-50.2544, 73.5706) (-50.8752, 74.3324) (-51.891, 74.3324) (-52.9069, 74.3324) (-53.5276, 73.5706) (-53.5276, 72.7028) (-53.5276, 71.8422) (-52.9069, 71.0804) (-51.891, 71.0804) (-50.8752, 71.0804) (-50.2544, 71.8422) (-50.2544, 72.7028) knots 0 0 0 0 1 1 1 2 2 2 3 3 3 4 4 4 4
  line L223 (-50.2544, 72.7028) -> (-50.2544, 73.5706) construction
  line L224 (-50.2544, 73.5706) -> (-50.8752, 74.3324) construction
  line L225 (-50.8752, 74.3324) -> (-51.891, 74.3324) construction
  line L226 (-51.891, 74.3324) -> (-52.9069, 74.3324) construction
  line L227 (-52.9069, 74.3324) -> (-53.5276, 73.5706) construction
  line L228 (-53.5276, 73.5706) -> (-53.5276, 72.7028) construction
  line L229 (-53.5276, 72.7028) -> (-53.5276, 71.8422) construction
  line L230 (-53.5276, 71.8422) -> (-52.9069, 71.0804) construction
  line L231 (-52.9069, 71.0804) -> (-51.891, 71.0804) construction
  line L232 (-51.891, 71.0804) -> (-50.8752, 71.0804) construction
  line L233 (-50.8752, 71.0804) -> (-50.2544, 71.8422) construction
  line L234 (-50.2544, 71.8422) -> (-50.2544, 72.7028) construction
  line L235 (-49.5208, 79.8781) -> (-49.5208, 79.8498)
  spline S30 degree 3 poles (-49.5208, 79.8498) (-49.5208, 79.6099) (-49.6266, 79.4547) (-49.8735, 79.2785) knots 1 1 1 1 2 2 2 2
  line L236 (-49.5208, 79.8498) -> (-49.5208, 79.6099) construction
  line L237 (-49.5208, 79.6099) -> (-49.6266, 79.4547) construction
  line L238 (-49.6266, 79.4547) -> (-49.8735, 79.2785) construction
  line L239 (-49.8735, 79.2785) -> (-53.0268, 77.0281)
  line L240 (-53.0268, 77.0281) -> (-49.8664, 77.0281)
  spline S31 degree 3 poles (-49.8664, 77.0281) (-49.6619, 77.0281) (-49.5208, 76.8659) (-49.5208, 76.64) (-49.5208, 76.4144) (-49.6619, 76.2521) (-49.8664, 76.2521) knots 4 4 4 4 5 5 5 6 6 6 6
  line L241 (-49.8664, 77.0281) -> (-49.6619, 77.0281) construction
  line L242 (-49.6619, 77.0281) -> (-49.5208, 76.8659) construction
  line L243 (-49.5208, 76.8659) -> (-49.5208, 76.64) construction
  line L244 (-49.5208, 76.64) -> (-49.5208, 76.4144) construction
  line L245 (-49.5208, 76.4144) -> (-49.6619, 76.2521) construction
  line L246 (-49.6619, 76.2521) -> (-49.8664, 76.2521) construction
  line L247 (-49.8664, 76.2521) -> (-53.7887, 76.2521)
  spline S32 degree 3 poles (-53.7887, 76.2521) (-54.0708, 76.2521) (-54.2543, 76.4425) (-54.2543, 76.6824) knots 7 7 7 7 8 8 8 8
  line L248 (-53.7887, 76.2521) -> (-54.0708, 76.2521) construction
  line L249 (-54.0708, 76.2521) -> (-54.2543, 76.4425) construction
  line L250 (-54.2543, 76.4425) -> (-54.2543, 76.6824) construction
  line L251 (-54.2543, 76.6824) -> (-54.2543, 76.7248)
  spline S33 degree 3 poles (-54.2543, 76.7248) (-54.2543, 76.9646) (-54.1696, 77.0915) (-53.8663, 77.3174) knots 9 9 9 9 10 10 10 10
  line L252 (-54.2543, 76.7248) -> (-54.2543, 76.9646) construction
  line L253 (-54.2543, 76.9646) -> (-54.1696, 77.0915) construction
  line L254 (-54.1696, 77.0915) -> (-53.8663, 77.3174) construction
  line L255 (-53.8663, 77.3174) -> (-50.8047, 79.5677)
  line L256 (-50.8047, 79.5677) -> (-53.9156, 79.5677)
  spline S34 degree 3 poles (-53.9156, 79.5677) (-54.1203, 79.5677) (-54.2613, 79.73) (-54.2613, 79.9556) (-54.2613, 80.1814) (-54.1203, 80.3437) (-53.9156, 80.3437) knots 12 12 12 12 13 13 13 14 14 14 14
  line L257 (-53.9156, 79.5677) -> (-54.1203, 79.5677) construction
  line L258 (-54.1203, 79.5677) -> (-54.2613, 79.73) construction
  line L259 (-54.2613, 79.73) -> (-54.2613, 79.9556) construction
  line L260 (-54.2613, 79.9556) -> (-54.2613, 80.1814) construction
  line L261 (-54.2613, 80.1814) -> (-54.1203, 80.3437) construction
  line L262 (-54.1203, 80.3437) -> (-53.9156, 80.3437) construction
  line L263 (-53.9156, 80.3437) -> (-49.937, 80.3437)
  spline S35 degree 3 poles (-49.937, 80.3437) (-49.69, 80.3437) (-49.5208, 80.1249) (-49.5208, 79.8781) knots 15 15 15 15 16 16 16 16
  line L264 (-49.937, 80.3437) -> (-49.69, 80.3437) construction
  line L265 (-49.69, 80.3437) -> (-49.5208, 80.1249) construction
  line L266 (-49.5208, 80.1249) -> (-49.5208, 79.8781) construction
  spline S36 degree 3 poles (-51.8981, 81.4167) (-53.2878, 81.4167) (-54.2895, 82.489) (-54.2895, 83.8858) (-54.2895, 85.2824) (-53.2878, 86.3618) (-51.8981, 86.3618) (-50.5014, 86.3618) (-49.4925, 85.2824) (-49.4925, 83.8858) (-49.4925, 82.489) (-50.5014, 81.4167) (-51.8981, 81.4167) knots 0 0 0 0 1 1 1 2 2 2 3 3 3 4 4 4 4
  line L267 (-51.8981, 81.4167) -> (-53.2878, 81.4167) construction
  line L268 (-53.2878, 81.4167) -> (-54.2895, 82.489) construction
  line L269 (-54.2895, 82.489) -> (-54.2895, 83.8858) construction
  line L270 (-54.2895, 83.8858) -> (-54.2895, 85.2824) construction
  line L271 (-54.2895, 85.2824) -> (-53.2878, 86.3618) construction
  line L272 (-53.2878, 86.3618) -> (-51.8981, 86.3618) construction
  line L273 (-51.8981, 86.3618) -> (-50.5014, 86.3618) construction
  line L274 (-50.5014, 86.3618) -> (-49.4925, 85.2824) construction
  line L275 (-49.4925, 85.2824) -> (-49.4925, 83.8858) construction
  line L276 (-49.4925, 83.8858) -> (-49.4925, 82.489) construction
  line L277 (-49.4925, 82.489) -> (-50.5014, 81.4167) construction
  line L278 (-50.5014, 81.4167) -> (-51.8981, 81.4167) construction
  spline S37 degree 3 poles (-50.2544, 83.8858) (-50.2544, 84.7534) (-50.8752, 85.5153) (-51.891, 85.5153) (-52.9069, 85.5153) (-53.5276, 84.7534) (-53.5276, 83.8858) (-53.5276, 83.025) (-52.9069, 82.2633) (-51.891, 82.2633) (-50.8752, 82.2633) (-50.2544, 83.025) (-50.2544, 83.8858) knots 0 0 0 0 1 1 1 2 2 2 3 3 3 4 4 4 4
  line L279 (-50.2544, 83.8858) -> (-50.2544, 84.7534) construction
  line L280 (-50.2544, 84.7534) -> (-50.8752, 85.5153) construction
  line L281 (-50.8752, 85.5153) -> (-51.891, 85.5153) construction
  line L282 (-51.891, 85.5153) -> (-52.9069, 85.5153) construction
  line L283 (-52.9069, 85.5153) -> (-53.5276, 84.7534) construction
  line L284 (-53.5276, 84.7534) -> (-53.5276, 83.8858) construction
  line L285 (-53.5276, 83.8858) -> (-53.5276, 83.025) construction
  line L286 (-53.5276, 83.025) -> (-52.9069, 82.2633) construction
  line L287 (-52.9069, 82.2633) -> (-51.891, 82.2633) construction
  line L288 (-51.891, 82.2633) -> (-50.8752, 82.2633) construction
  line L289 (-50.8752, 82.2633) -> (-50.2544, 83.025) construction
  line L290 (-50.2544, 83.025) -> (-50.2544, 83.8858) construction
  line L291 (-53.0127, 91.1456) -> (-51.5242, 90.1297)
  spline S38 degree 3 poles (-51.5242, 90.1297) (-51.3126, 89.9886) (-51.2279, 89.8758) (-51.2279, 89.6852) (-51.2279, 89.5018) (-51.3126, 89.396) (-51.5242, 89.2479) knots 1 1 1 1 2 2 2 3 3 3 3
  line L292 (-51.5242, 90.1297) -> (-51.3126, 89.9886) construction
  line L293 (-51.3126, 89.9886) -> (-51.2279, 89.8758) construction
  line L294 (-51.2279, 89.8758) -> (-51.2279, 89.6852) construction
  line L295 (-51.2279, 89.6852) -> (-51.2279, 89.5018) construction
  line L296 (-51.2279, 89.5018) -> (-51.3126, 89.396) construction
  line L297 (-51.3126, 89.396) -> (-51.5242, 89.2479) construction
  line L298 (-51.5242, 89.2479) -> (-53.0127, 88.2321)
  line L299 (-53.0127, 88.2321) -> (-53.0127, 88.2109)
  line L300 (-53.0127, 88.2109) -> (-49.8664, 88.2109)
  spline S39 degree 3 poles (-49.8664, 88.2109) (-49.6548, 88.2109) (-49.5208, 88.0487) (-49.5208, 87.823) (-49.5208, 87.5972) (-49.6548, 87.4349) (-49.8664, 87.4349) knots 6 6 6 6 7 7 7 8 8 8 8
  line L301 (-49.8664, 88.2109) -> (-49.6548, 88.2109) construction
  line L302 (-49.6548, 88.2109) -> (-49.5208, 88.0487) construction
  line L303 (-49.5208, 88.0487) -> (-49.5208, 87.823) construction
  line L304 (-49.5208, 87.823) -> (-49.5208, 87.5972) construction
  line L305 (-49.5208, 87.5972) -> (-49.6548, 87.4349) construction
  line L306 (-49.6548, 87.4349) -> (-49.8664, 87.4349) construction
  line L307 (-49.8664, 87.4349) -> (-53.8028, 87.4349)
  spline S40 degree 3 poles (-53.8028, 87.4349) (-54.0779, 87.4349) (-54.2543, 87.6325) (-54.2543, 87.8935) knots 9 9 9 9 10 10 10 10
  line L308 (-53.8028, 87.4349) -> (-54.0779, 87.4349) construction
  line L309 (-54.0779, 87.4349) -> (-54.2543, 87.6325) construction
  line L310 (-54.2543, 87.6325) -> (-54.2543, 87.8935) construction
  line L311 (-54.2543, 87.8935) -> (-54.2543, 87.95)
  spline S41 degree 3 poles (-54.2543, 87.95) (-54.2543, 88.218) (-54.092, 88.3873) (-53.8804, 88.5284) knots 11 11 11 11 12 12 12 12
  line L312 (-54.2543, 87.95) -> (-54.2543, 88.218) construction
  line L313 (-54.2543, 88.218) -> (-54.092, 88.3873) construction
  line L314 (-54.092, 88.3873) -> (-53.8804, 88.5284) construction
  line L315 (-53.8804, 88.5284) -> (-52.1591, 89.7064)
  line L316 (-52.1591, 89.7064) -> (-52.1591, 89.7135)
  line L317 (-52.1591, 89.7135) -> (-53.8875, 90.8847)
  spline S42 degree 3 poles (-53.8875, 90.8847) (-54.092, 91.0257) (-54.2543, 91.1597) (-54.2543, 91.4278) knots 15 15 15 15 16 16 16 16
  line L318 (-53.8875, 90.8847) -> (-54.092, 91.0257) construction
  line L319 (-54.092, 91.0257) -> (-54.2543, 91.1597) construction
  line L320 (-54.2543, 91.1597) -> (-54.2543, 91.4278) construction
  line L321 (-54.2543, 91.4278) -> (-54.2543, 91.4843)
  spline S43 degree 3 poles (-54.2543, 91.4843) (-54.2543, 91.7382) (-54.0779, 91.9358) (-53.8028, 91.9358) knots 17 17 17 17 18 18 18 18
  line L322 (-54.2543, 91.4843) -> (-54.2543, 91.7382) construction
  line L323 (-54.2543, 91.7382) -> (-54.0779, 91.9358) construction
  line L324 (-54.0779, 91.9358) -> (-53.8028, 91.9358) construction
  line L325 (-53.8028, 91.9358) -> (-49.8664, 91.9358)
  spline S44 degree 3 poles (-49.8664, 91.9358) (-49.6548, 91.9358) (-49.5208, 91.7735) (-49.5208, 91.5477) (-49.5208, 91.322) (-49.6548, 91.1597) (-49.8664, 91.1597) knots 19 19 19 19 20 20 20 21 21 21 21
  line L326 (-49.8664, 91.9358) -> (-49.6548, 91.9358) construction
  line L327 (-49.6548, 91.9358) -> (-49.5208, 91.7735) construction
  line L328 (-49.5208, 91.7735) -> (-49.5208, 91.5477) construction
  line L329 (-49.5208, 91.5477) -> (-49.5208, 91.322) construction
  line L330 (-49.5208, 91.322) -> (-49.6548, 91.1597) construction
  line L331 (-49.6548, 91.1597) -> (-49.8664, 91.1597) construction
  line L332 (-49.8664, 91.1597) -> (-53.0127, 91.1597)
  line L333 (-53.0127, 91.1597) -> (-53.0127, 91.1456)
  spline S45 degree 3 poles (-51.8981, 93.0089) (-53.2878, 93.0089) (-54.2895, 94.0812) (-54.2895, 95.478) (-54.2895, 96.8748) (-53.2878, 97.9542) (-51.8981, 97.9542) (-50.5014, 97.9542) (-49.4925, 96.8748) (-49.4925, 95.478) (-49.4925, 94.0812) (-50.5014, 93.0089) (-51.8981, 93.0089) knots 0 0 0 0 1 1 1 2 2 2 3 3 3 4 4 4 4
  line L334 (-51.8981, 93.0089) -> (-53.2878, 93.0089) construction
  line L335 (-53.2878, 93.0089) -> (-54.2895, 94.0812) construction
  line L336 (-54.2895, 94.0812) -> (-54.2895, 95.478) construction
  line L337 (-54.2895, 95.478) -> (-54.2895, 96.8748) construction
  line L338 (-54.2895, 96.8748) -> (-53.2878, 97.9542) construction
  line L339 (-53.2878, 97.9542) -> (-51.8981, 97.9542) construction
  line L340 (-51.8981, 97.9542) -> (-50.5014, 97.9542) construction
  line L341 (-50.5014, 97.9542) -> (-49.4925, 96.8748) construction
  line L342 (-49.4925, 96.8748) -> (-49.4925, 95.478) construction
  line L343 (-49.4925, 95.478) -> (-49.4925, 94.0812) construction
  line L344 (-49.4925, 94.0812) -> (-50.5014, 93.0089) construction
  line L345 (-50.5014, 93.0089) -> (-51.8981, 93.0089) construction
  spline S46 degree 3 poles (-50.2544, 95.478) (-50.2544, 96.3456) (-50.8752, 97.1075) (-51.891, 97.1075) (-52.9069, 97.1075) (-53.5276, 96.3456) (-53.5276, 95.478) (-53.5276, 94.6174) (-52.9069, 93.8555) (-51.891, 93.8555) (-50.8752, 93.8555) (-50.2544, 94.6174) (-50.2544, 95.478) knots 0 0 0 0 1 1 1 2 2 2 3 3 3 4 4 4 4
  line L346 (-50.2544, 95.478) -> (-50.2544, 96.3456) construction
  line L347 (-50.2544, 96.3456) -> (-50.8752, 97.1075) construction
  line L348 (-50.8752, 97.1075) -> (-51.891, 97.1075) construction
  line L349 (-51.891, 97.1075) -> (-52.9069, 97.1075) construction
  line L350 (-52.9069, 97.1075) -> (-53.5276, 96.3456) construction
  line L351 (-53.5276, 96.3456) -> (-53.5276, 95.478) construction
  line L352 (-53.5276, 95.478) -> (-53.5276, 94.6174) construction
  line L353 (-53.5276, 94.6174) -> (-52.9069, 93.8555) construction
  line L354 (-52.9069, 93.8555) -> (-51.891, 93.8555) construction
  line L355 (-51.891, 93.8555) -> (-50.8752, 93.8555) construction
  line L356 (-50.8752, 93.8555) -> (-50.2544, 94.6174) construction
  line L357 (-50.2544, 94.6174) -> (-50.2544, 95.478) construction
  spline S47 degree 3 poles (-50.2332, 100.9883) (-50.2332, 101.7431) (-50.7482, 102.2157) (-51.5525, 102.2157) knots 0 0 0 0 1 1 1 1
  line L358 (-50.2332, 100.9883) -> (-50.2332, 101.7431) construction
  line L359 (-50.2332, 101.7431) -> (-50.7482, 102.2157) construction
  line L360 (-50.7482, 102.2157) -> (-51.5525, 102.2157) construction
  line L361 (-51.5525, 102.2157) -> (-53.9156, 102.2157)
  spline S48 degree 3 poles (-53.9156, 102.2157) (-54.1203, 102.2157) (-54.2613, 102.378) (-54.2613, 102.6038) (-54.2613, 102.8295) (-54.1203, 102.9918) (-53.9156, 102.9918) knots 2 2 2 2 3 3 3 4 4 4 4
  line L362 (-53.9156, 102.2157) -> (-54.1203, 102.2157) construction
  line L363 (-54.1203, 102.2157) -> (-54.2613, 102.378) construction
  line L364 (-54.2613, 102.378) -> (-54.2613, 102.6038) construction
  line L365 (-54.2613, 102.6038) -> (-54.2613, 102.8295) construction
  line L366 (-54.2613, 102.8295) -> (-54.1203, 102.9918) construction
  line L367 (-54.1203, 102.9918) -> (-53.9156, 102.9918) construction
  line L368 (-53.9156, 102.9918) -> (-51.5101, 102.9918)
  spline S49 degree 3 poles (-51.5101, 102.9918) (-50.3391, 102.9918) (-49.4784, 102.244) (-49.4784, 100.9883) (-49.4784, 99.7256) (-50.3391, 98.9849) (-51.5101, 98.9849) knots 5 5 5 5 6 6 6 7 7 7 7
  line L369 (-51.5101, 102.9918) -> (-50.3391, 102.9918) construction
  line L370 (-50.3391, 102.9918) -> (-49.4784, 102.244) construction
  line L371 (-49.4784, 102.244) -> (-49.4784, 100.9883) construction
  line L372 (-49.4784, 100.9883) -> (-49.4784, 99.7256) construction
  line L373 (-49.4784, 99.7256) -> (-50.3391, 98.9849) construction
  line L374 (-50.3391, 98.9849) -> (-51.5101, 98.9849) construction
  line L375 (-51.5101, 98.9849) -> (-53.9156, 98.9849)
  spline S50 degree 3 poles (-53.9156, 98.9849) (-54.1203, 98.9849) (-54.2613, 99.1472) (-54.2613, 99.3729) (-54.2613, 99.5987) (-54.1203, 99.7609) (-53.9156, 99.7609) knots 8 8 8 8 9 9 9 10 10 10 10
  line L376 (-53.9156, 98.9849) -> (-54.1203, 98.9849) construction
  line L377 (-54.1203, 98.9849) -> (-54.2613, 99.1472) construction
  line L378 (-54.2613, 99.1472) -> (-54.2613, 99.3729) construction
  line L379 (-54.2613, 99.3729) -> (-54.2613, 99.5987) construction
  line L380 (-54.2613, 99.5987) -> (-54.1203, 99.7609) construction
  line L381 (-54.1203, 99.7609) -> (-53.9156, 99.7609) construction
  line L382 (-53.9156, 99.7609) -> (-51.5525, 99.7609)
  spline S51 degree 3 poles (-51.5525, 99.7609) (-50.7553, 99.7609) (-50.2332, 100.2264) (-50.2332, 100.9883) knots 11 11 11 11 12 12 12 12
  line L383 (-51.5525, 99.7609) -> (-50.7553, 99.7609) construction
  line L384 (-50.7553, 99.7609) -> (-50.2332, 100.2264) construction
  line L385 (-50.2332, 100.2264) -> (-50.2332, 100.9883) construction
  spline S52 degree 3 poles (-53.9156, 107.5427) (-53.838, 107.6697) (-53.7393, 107.7966) (-53.5771, 107.7966) (-53.3865, 107.7966) (-53.1961, 107.6767) (-53.1961, 107.4581) (-53.1961, 107.3452) (-53.2243, 107.2747) (-53.2808, 107.1689) (-53.4219, 106.8725) (-53.5559, 106.4704) (-53.5559, 106.0401) (-53.5559, 105.363) (-53.2455, 104.989) (-52.8928, 104.989) (-52.4201, 104.989) (-52.3002, 105.4476) (-52.138, 106.2799) (-51.9686, 107.1336) (-51.7853, 107.9096) (-50.8399, 107.9096) (-50.0992, 107.9096) (-49.4855, 107.2111) (-49.4855, 106.0543) (-49.4855, 105.3065) (-49.7183, 104.6082) (-49.9582, 104.2413) (-50.0569, 104.1002) (-50.1839, 104.0649) (-50.2756, 104.0649) (-50.4802, 104.0649) (-50.6777, 104.2201) (-50.6777, 104.4247) (-50.6777, 104.5234) (-50.6354, 104.6221) (-50.5859, 104.721) (-50.3884, 105.116) (-50.2403, 105.5957) (-50.2403, 106.0966) (-50.2403, 106.7385) (-50.4731, 107.0842) (-50.8258, 107.0842) (-51.2138, 107.0842) (-51.3126, 106.7104) (-51.4819, 105.8567) (-51.6512, 104.9961) (-51.8417, 104.1636) (-52.8786, 104.1636) (-53.5982, 104.1636) (-54.2895, 104.8197) (-54.2895, 106.0755) (-54.2895, 106.7033) (-54.0638, 107.2959) (-53.9156, 107.5427) knots 0 0 0 0 1 1 1 2 2 2 3 3 3 4 4 4 5 5 5 6 6 6 7 7 7 8 8 8 9 9 9 10 10 10 11 11 11 12 12 12 13 13 13 14 14 14 15 15 15 16 16 16 17 17 17 18 18 18 18
  line L386 (-53.9156, 107.5427) -> (-53.838, 107.6697) construction
  line L387 (-53.838, 107.6697) -> (-53.7393, 107.7966) construction
  line L388 (-53.7393, 107.7966) -> (-53.5771, 107.7966) construction
  line L389 (-53.5771, 107.7966) -> (-53.3865, 107.7966) construction
  line L390 (-53.3865, 107.7966) -> (-53.1961, 107.6767) construction
  line L391 (-53.1961, 107.6767) -> (-53.1961, 107.4581) construction
  line L392 (-53.1961, 107.4581) -> (-53.1961, 107.3452) construction
  line L393 (-53.1961, 107.3452) -> (-53.2243, 107.2747) construction
  line L394 (-53.2243, 107.2747) -> (-53.2808, 107.1689) construction
  line L395 (-53.2808, 107.1689) -> (-53.4219, 106.8725) construction
  line L396 (-53.4219, 106.8725) -> (-53.5559, 106.4704) construction
  line L397 (-53.5559, 106.4704) -> (-53.5559, 106.0401) construction
  line L398 (-53.5559, 106.0401) -> (-53.5559, 105.363) construction
  line L399 (-53.5559, 105.363) -> (-53.2455, 104.989) construction
  line L400 (-53.2455, 104.989) -> (-52.8928, 104.989) construction
  line L401 (-52.8928, 104.989) -> (-52.4201, 104.989) construction
  line L402 (-52.4201, 104.989) -> (-52.3002, 105.4476) construction
  line L403 (-52.3002, 105.4476) -> (-52.138, 106.2799) construction
  line L404 (-52.138, 106.2799) -> (-51.9686, 107.1336) construction
  line L405 (-51.9686, 107.1336) -> (-51.7853, 107.9096) construction
  line L406 (-51.7853, 107.9096) -> (-50.8399, 107.9096) construction